Autodesk Fusion 360 part; units mm, degrees
(part 4 of 9)
  line L470 (39.3109, 74.8923) -> (43.641, 72.3923)
  line L471 (43.641, 72.3923) -> (47.9711, 74.8923)
  line L472 (47.9711, 74.8923) -> (47.9711, 79.8923)
  line L473 (47.9711, 79.8923) -> (43.641, 82.3923)
  line L474 (53.8013, 82.3923) -> (49.4711, 79.8923)
  line L475 (49.4711, 79.8923) -> (49.4711, 74.8923)
  line L476 (49.4711, 74.8923) -> (53.8013, 72.3923)
  line L477 (53.8013, 72.3923) -> (58.1314, 74.8923)
  line L478 (58.1314, 74.8923) -> (58.1314, 79.8923)
  line L479 (58.1314, 79.8923) -> (53.8013, 82.3923)
  line L480 (63.9615, 82.3923) -> (59.6314, 79.8923)
  line L481 (59.6314, 79.8923) -> (59.6314, 74.8923)
  line L482 (59.6314, 74.8923) -> (63.9615, 72.3923)
  line L483 (63.9615, 72.3923) -> (68.2917, 74.8923)
  line L484 (68.2917, 74.8923) -> (68.2917, 79.8923)
  line L485 (68.2917, 79.8923) -> (63.9615, 82.3923)
  line L486 (74.1218, 82.3923) -> (69.7917, 79.8923)
  line L487 (69.7917, 79.8923) -> (69.7917, 74.8923)
  line L488 (69.7917, 74.8923) -> (74.1218, 72.3923)
  line L489 (74.1218, 72.3923) -> (78.4519, 74.8923)
  line L490 (78.4519, 74.8923) -> (78.4519, 79.8923)
  line L491 (78.4519, 79.8923) -> (74.1218, 82.3923)
  line L492 (84.282, 82.3923) -> (79.9519, 79.8923)
  line L493 (79.9519, 79.8923) -> (79.9519, 74.8923)
  line L494 (79.9519, 74.8923) -> (84.282, 72.3923)
  line L495 (84.282, 72.3923) -> (88.6122, 74.8923)
  line L496 (88.6122, 74.8923) -> (88.6122, 79.8923)
  line L497 (88.6122, 79.8923) -> (84.282, 82.3923)
  line L498 (94.4423, 82.3923) -> (90.1122, 79.8923)
  line L499 (90.1122, 79.8923) -> (90.1122, 74.8923)
  line L500 (90.1122, 74.8923) -> (94.4423, 72.3923)
  line L501 (94.4423, 72.3923) -> (98.7724, 74.8923)
  line L502 (98.7724, 74.8923) -> (98.7724, 79.8923)
  line L503 (98.7724, 79.8923) -> (94.4423, 82.3923)
  line L504 (104.6025, 82.3923) -> (100.2724, 79.8923)
  line L505 (100.2724, 79.8923) -> (100.2724, 74.8923)
  line L506 (100.2724, 74.8923) -> (104.6025, 72.3923)
  line L507 (104.6025, 72.3923) -> (108.9327, 74.8923)
  line L508 (108.9327, 74.8923) -> (108.9327, 79.8923)
  line L509 (108.9327, 79.8923) -> (104.6025, 82.3923)
  line L510 (8.0801, 91.1913) -> (3.75, 88.6913)
  line L511 (3.75, 88.6913) -> (3.75, 83.6913)
  line L512 (3.75, 83.6913) -> (8.0801, 81.1913)
  line L513 (8.0801, 81.1913) -> (12.4103, 83.6913)
  line L514 (12.4103, 83.6913) -> (12.4103, 88.6913)
  line L515 (12.4103, 88.6913) -> (8.0801, 91.1913)
  line L516 (18.2404, 91.1913) -> (13.9103, 88.6913)
  line L517 (13.9103, 88.6913) -> (13.9103, 83.6913)
  line L518 (13.9103, 83.6913) -> (18.2404, 81.1913)
  line L519 (18.2404, 81.1913) -> (22.5705, 83.6913)
  line L520 (22.5705, 83.6913) -> (22.5705, 88.6913)
  line L521 (22.5705, 88.6913) -> (18.2404, 91.1913)
  line L522 (28.4006, 91.1913) -> (24.0705, 88.6913)
  line L523 (24.0705, 88.6913) -> (24.0705, 83.6913)
  line L524 (24.0705, 83.6913) -> (28.4006, 81.1913)
  line L525 (28.4006, 81.1913) -> (32.7308, 83.6913)
  line L526 (32.7308, 83.6913) -> (32.7308, 88.6913)
  line L527 (32.7308, 88.6913) -> (28.4006, 91.1913)
  line L528 (38.5609, 91.1913) -> (34.2308, 88.6913)
  line L529 (34.2308, 88.6913) -> (34.2308, 83.6913)
  line L530 (34.2308, 83.6913) -> (38.5609, 81.1913)
  line L531 (38.5609, 81.1913) -> (42.891, 83.6913)
  line L532 (42.891, 83.6913) -> (42.891, 88.6913)
  line L533 (42.891, 88.6913) -> (38.5609, 91.1913)
  line L534 (48.7211, 91.1913) -> (44.391, 88.6913)
  line L535 (44.391, 88.6913) -> (44.391, 83.6913)
  line L536 (44.391, 83.6913) -> (48.7211, 81.1913)
  line L537 (48.7211, 81.1913) -> (53.0513, 83.6913)
  line L538 (53.0513, 83.6913) -> (53.0513, 88.6913)
  line L539 (53.0513, 88.6913) -> (48.7211, 91.1913)
  line L540 (58.8814, 91.1913) -> (54.5513, 88.6913)
  line L541 (54.5513, 88.6913) -> (54.5513, 83.6913)
  line L542 (54.5513, 83.6913) -> (58.8814, 81.1913)
  line L543 (58.8814, 81.1913) -> (63.2115, 83.6913)
  line L544 (63.2115, 83.6913) -> (63.2115, 88.6913)
  line L545 (63.2115, 88.6913) -> (58.8814, 91.1913)
  line L546 (69.0417, 91.1913) -> (64.7115, 88.6913)
  line L547 (64.7115, 88.6913) -> (64.7115, 83.6913)
  line L548 (64.7115, 83.6913) -> (69.0417, 81.1913)
  line L549 (69.0417, 81.1913) -> (73.3718, 83.6913)
  line L550 (73.3718, 83.6913) -> (73.3718, 88.6913)
  line L551 (73.3718, 88.6913) -> (69.0417, 91.1913)
  line L552 (79.2019, 91.1913) -> (74.8718, 88.6913)
  line L553 (74.8718, 88.6913) -> (74.8718, 83.6913)
  line L554 (74.8718, 83.6913) -> (79.2019, 81.1913)
  line L555 (79.2019, 81.1913) -> (83.532, 83.6913)
  line L556 (83.532, 83.6913) -> (83.532, 88.6913)
  line L557 (83.532, 88.6913) -> (79.2019, 91.1913)
  line L558 (89.3622, 91.1913) -> (85.032, 88.6913)
  line L559 (85.032, 88.6913) -> (85.032, 83.6913)
  line L560 (85.032, 83.6913) -> (89.3622, 81.1913)
  line L561 (89.3622, 81.1913) -> (93.6923, 83.6913)
  line L562 (93.6923, 83.6913) -> (93.6923, 88.6913)
  line L563 (93.6923, 88.6913) -> (89.3622, 91.1913)
  line L564 (99.5224, 91.1913) -> (95.1923, 88.6913)
  line L565 (95.1923, 88.6913) -> (95.1923, 83.6913)
  line L566 (95.1923, 83.6913) -> (99.5224, 81.1913)
  line L567 (99.5224, 81.1913) -> (103.8525, 83.6913)
  line L568 (103.8525, 83.6913) -> (103.8525, 88.6913)
  line L569 (103.8525, 88.6913) -> (99.5224, 91.1913)
  line L570 (3, 99.9904) -> (-1.3301, 97.4904)
  line L571 (-1.3301, 97.4904) -> (-1.3301, 92.4904)
  line L572 (-1.3301, 92.4904) -> (3, 89.9904)
  line L573 (3, 89.9904) -> (7.3301, 92.4904)
  line L574 (7.3301, 92.4904) -> (7.3301, 97.4904)
  line L575 (7.3301, 97.4904) -> (3, 99.9904)
  line L576 (13.1603, 99.9904) -> (8.8301, 97.4904)
  line L577 (8.8301, 97.4904) -> (8.8301, 92.4904)
  line L578 (8.8301, 92.4904) -> (13.1603, 89.9904)
  line L579 (13.1603, 89.9904) -> (17.4904, 92.4904)
  line L580 (17.4904, 92.4904) -> (17.4904, 97.4904)
  line L581 (17.4904, 97.4904) -> (13.1603, 99.9904)
  line L582 (23.3205, 99.9904) -> (18.9904, 97.4904)
  line L583 (18.9904, 97.4904) -> (18.9904, 92.4904)
  line L584 (18.9904, 92.4904) -> (23.3205, 89.9904)
  line L585 (23.3205, 89.9904) -> (27.6506, 92.4904)
  line L586 (27.6506, 92.4904) -> (27.6506, 97.4904)
  line L587 (27.6506, 97.4904) -> (23.3205, 99.9904)
  line L588 (33.4808, 99.9904) -> (29.1506, 97.4904)
  line L589 (29.1506, 97.4904) -> (29.1506, 92.4904)
  line L590 (29.1506, 92.4904) -> (33.4808, 89.9904)
  line L591 (33.4808, 89.9904) -> (37.8109, 92.4904)
  line L592 (37.8109, 92.4904) -> (37.8109, 97.4904)
  line L593 (37.8109, 97.4904) -> (33.4808, 99.9904)
  line L594 (43.641, 99.9904) -> (39.3109, 97.4904)
  line L595 (39.3109, 97.4904) -> (39.3109, 92.4904)
  line L596 (39.3109, 92.4904) -> (43.641, 89.9904)
  line L597 (43.641, 89.9904) -> (47.9711, 92.4904)
  line L598 (47.9711, 92.4904) -> (47.9711, 97.4904)
  line L599 (47.9711, 97.4904) -> (43.641, 99.9904)
  line L600 (53.8013, 99.9904) -> (49.4711, 97.4904)
  line L601 (49.4711, 97.4904) -> (49.4711, 92.4904)
  line L602 (49.4711, 92.4904) -> (53.8013, 89.9904)
  line L603 (53.8013, 89.9904) -> (58.1314, 92.4904)
  line L604 (58.1314, 92.4904) -> (58.1314, 97.4904)
  line L605 (58.1314, 97.4904) -> (53.8013, 99.9904)
  line L606 (63.9615, 99.9904) -> (59.6314, 97.4904)
  line L607 (59.6314, 97.4904) -> (59.6314, 92.4904)
  line L608 (59.6314, 92.4904) -> (63.9615, 89.9904)
  line L609 (63.9615, 89.9904) -> (68.2917, 92.4904)
  line L610 (68.2917, 92.4904) -> (68.2917, 97.4904)
  line L611 (68.2917, 97.4904) -> (63.9615, 99.9904)
  line L612 (74.1218, 99.9904) -> (69.7917, 97.4904)
  line L613 (69.7917, 97.4904) -> (69.7917, 92.4904)
  line L614 (69.7917, 92.4904) -> (74.1218, 89.9904)
  line L615 (74.1218, 89.9904) -> (78.4519, 92.4904)
  line L616 (78.4519, 92.4904) -> (78.4519, 97.4904)
  line L617 (78.4519, 97.4904) -> (74.1218, 99.9904)
  line L618 (84.282, 99.9904) -> (79.9519, 97.4904)
  line L619 (79.9519, 97.4904) -> (79.9519, 92.4904)
  line L620 (79.9519, 92.4904) -> (84.282, 89.9904)
  line L621 (84.282, 89.9904) -> (88.6122, 92.4904)
  line L622 (88.6122, 92.4904) -> (88.6122, 97.4904)
  line L623 (88.6122, 97.4904) -> (84.282, 99.9904)
  line L624 (94.4423, 99.9904) -> (90.1122, 97.4904)
  line L625 (90.1122, 97.4904) -> (90.1122, 92.4904)
  line L626 (90.1122, 92.4904) -> (94.4423, 89.9904)
  line L627 (94.4423, 89.9904) -> (98.7724, 92.4904)
  line L628 (98.7724, 92.4904) -> (98.7724, 97.4904)
  line L629 (98.7724, 97.4904) -> (94.4423, 99.9904)
  line L630 (104.6025, 99.9904) -> (100.2724, 97.4904)
  line L631 (100.2724, 97.4904) -> (100.2724, 92.4904)
  line L632 (100.2724, 92.4904) -> (104.6025, 89.9904)
  line L633 (104.6025, 89.9904) -> (108.9327, 92.4904)
  line L634 (108.9327, 92.4904) -> (108.9327, 97.4904)
  line L635 (108.9327, 97.4904) -> (104.6025, 99.9904)
  line L636 (8.0801, 108.7894) -> (3.75, 106.2894)
  line L637 (3.75, 106.2894) -> (3.75, 101.2894)
  line L638 (3.75, 101.2894) -> (8.0801, 98.7894)
  line L639 (8.0801, 98.7894) -> (12.4103, 101.2894)
  line L640 (12.4103, 101.2894) -> (12.4103, 106.2894)
  line L641 (12.4103, 106.2894) -> (8.0801, 108.7894)
  line L642 (18.2404, 108.7894) -> (13.9103, 106.2894)
  line L643 (13.9103, 106.2894) -> (13.9103, 101.2894)
  line L644 (13.9103, 101.2894) -> (18.2404, 98.7894)
  line L645 (18.2404, 98.7894) -> (22.5705, 101.2894)
  line L646 (22.5705, 101.2894) -> (22.5705, 106.2894)
  line L647 (22.5705, 106.2894) -> (18.2404, 108.7894)
  line L648 (28.4006, 108.7894) -> (24.0705, 106.2894)
  line L649 (24.0705, 106.2894) -> (24.0705, 101.2894)
  line L650 (24.0705, 101.2894) -> (28.4006, 98.7894)
  line L651 (28.4006, 98.7894) -> (32.7308, 101.2894)
  line L652 (32.7308, 101.2894) -> (32.7308, 106.2894)
  line L653 (32.7308, 106.2894) -> (28.4006, 108.7894)
  line L654 (38.5609, 108.7894) -> (34.2308, 106.2894)
  line L655 (34.2308, 106.2894) -> (34.2308, 101.2894)
  line L656 (34.2308, 101.2894) -> (38.5609, 98.7894)
  line L657 (38.5609, 98.7894) -> (42.891, 101.2894)
  line L658 (42.891, 101.2894) -> (42.891, 106.2894)
  line L659 (42.891, 106.2894) -> (38.5609, 108.7894)
  line L660 (48.7211, 108.7894) -> (44.391, 106.2894)
  line L661 (44.391, 106.2894) -> (44.391, 101.2894)
  line L662 (44.391, 101.2894) -> (48.7211, 98.7894)
  line L663 (48.7211, 98.7894) -> (53.0513, 101.2894)
  line L664 (53.0513, 101.2894) -> (53.0513, 106.2894)
  line L665 (53.0513, 106.2894) -> (48.7211, 108.7894)
  line L666 (58.8814, 108.7894) -> (54.5513, 106.2894)
  line L667 (54.5513, 106.2894) -> (54.5513, 101.2894)
  line L668 (54.5513, 101.2894) -> (58.8814, 98.7894)
  line L669 (58.8814, 98.7894) -> (63.2115, 101.2894)
  line L670 (63.2115, 101.2894) -> (63.2115, 106.2894)
  line L671 (63.2115, 106.2894) -> (58.8814, 108.7894)
  line L672 (69.0417, 108.7894) -> (64.7115, 106.2894)
  line L673 (64.7115, 106.2894) -> (64.7115, 101.2894)
  line L674 (64.7115, 101.2894) -> (69.0417, 98.7894)
  line L675 (69.0417, 98.7894) -> (73.3718, 101.2894)
  line L676 (73.3718, 101.2894) -> (73.3718, 106.2894)
  line L677 (73.3718, 106.2894) -> (69.0417, 108.7894)
  line L678 (79.2019, 108.7894) -> (74.8718, 106.2894)
  line L679 (74.8718, 106.2894) -> (74.8718, 101.2894)
  line L680 (74.8718, 101.2894) -> (79.2019, 98.7894)
  line L681 (79.2019, 98.7894) -> (83.532, 101.2894)
  line L682 (83.532, 101.2894) -> (83.532, 106.2894)
  line L683 (83.532, 106.2894) -> (79.2019, 108.7894)
  line L684 (89.3622, 108.7894) -> (85.032, 106.2894)
  line L685 (85.032, 106.2894) -> (85.032, 101.2894)
  line L686 (85.032, 101.2894) -> (89.3622, 98.7894)
  line L687 (89.3622, 98.7894) -> (93.6923, 101.2894)
  line L688 (93.6923, 101.2894) -> (93.6923, 106.2894)
  line L689 (93.6923, 106.2894) -> (89.3622, 108.7894)
  line L690 (99.5224, 108.7894) -> (95.1923, 106.2894)
  line L691 (95.1923, 106.2894) -> (95.1923, 101.2894)
  line L692 (95.1923, 101.2894) -> (99.5224, 98.7894)
  line L693 (99.5224, 98.7894) -> (103.8525, 101.2894)
  line L694 (103.8525, 101.2894) -> (103.8525, 106.2894)
  line L695 (103.8525, 106.2894) -> (99.5224, 108.7894)
  line L696 (3, 117.5885) -> (-1.3301, 115.0885)
  line L697 (-1.3301, 115.0885) -> (-1.3301, 110.0885)
  line L698 (-1.3301, 110.0885) -> (3, 107.5885)
  line L699 (3, 107.5885) -> (7.3301, 110.0885)
  line L700 (7.3301, 110.0885) -> (7.3301, 115.0885)
  line L701 (7.3301, 115.0885) -> (3, 117.5885)
  line L702 (13.1603, 117.5885) -> (8.8301, 115.0885)
  line L703 (8.8301, 115.0885) -> (8.8301, 110.0885)
  line L704 (8.8301, 110.0885) -> (13.1603, 107.5885)
  line L705 (13.1603, 107.5885) -> (17.4904, 110.0885)
  line L706 (17.4904, 110.0885) -> (17.4904, 115.0885)
  line L707 (17.4904, 115.0885) -> (13.1603, 117.5885)
  line L708 (23.3205, 117.5885) -> (18.9904, 115.0885)
  line L709 (18.9904, 115.0885) -> (18.9904, 110.0885)
  line L710 (18.9904, 110.0885) -> (23.3205, 107.5885)
  line L711 (23.3205, 107.5885) -> (27.6506, 110.0885)
  line L712 (27.6506, 110.0885) -> (27.6506, 115.0885)
  line L713 (27.6506, 115.0885) -> (23.3205, 117.5885)
  line L714 (33.4808, 117.5885) -> (29.1506, 115.0885)
  line L715 (29.1506, 115.0885) -> (29.1506, 110.0885)
  line L716 (29.1506, 110.0885) -> (33.4808, 107.5885)
  line L717 (33.4808, 107.5885) -> (37.8109, 110.0885)
  line L718 (37.8109, 110.0885) -> (37.8109, 115.0885)
  line L719 (37.8109, 115.0885) -> (33.4808, 117.5885)
  line L720 (43.641, 117.5885) -> (39.3109, 115.0885)
  line L721 (39.3109, 115.0885) -> (39.3109, 110.0885)
  line L722 (39.3109, 110.0885) -> (43.641, 107.5885)
  line L723 (43.641, 107.5885) -> (47.9711, 110.0885)
  line L724 (47.9711, 110.0885) -> (47.9711, 115.0885)
  line L725 (47.9711, 115.0885) -> (43.641, 117.5885)
  line L726 (53.8013, 117.5885) -> (49.4711, 115.0885)
  line L727 (49.4711, 115.0885) -> (49.4711, 110.0885)
  line L728 (49.4711, 110.0885) -> (53.8013, 107.5885)
  line L729 (53.8013, 107.5885) -> (58.1314, 110.0885)
  line L730 (58.1314, 110.0885) -> (58.1314, 115.0885)
  line L731 (58.1314, 115.0885) -> (53.8013, 117.5885)
  line L732 (63.9615, 117.5885) -> (59.6314, 115.0885)
  line L733 (59.6314, 115.0885) -> (59.6314, 110.0885)
  line L734 (59.6314, 110.0885) -> (63.9615, 107.5885)
  line L735 (63.9615, 107.5885) -> (68.2917, 110.0885)
  line L736 (68.2917, 110.0885) -> (68.2917, 115.0885)
  line L737 (68.2917, 115.0885) -> (63.9615, 117.5885)
  line L738 (74.1218, 117.5885) -> (69.7917, 115.0885)
  line L739 (69.7917, 115.0885) -> (69.7917, 110.0885)
  line L740 (69.7917, 110.0885) -> (74.1218, 107.5885)
  line L741 (74.1218, 107.5885) -> (78.4519, 110.0885)
  line L742 (78.4519, 110.0885) -> (78.4519, 115.0885)
  line L743 (78.4519, 115.0885) -> (74.1218, 117.5885)
  line L744 (84.282, 117.5885) -> (79.9519, 115.0885)
  line L745 (79.9519, 115.0885) -> (79.9519, 110.0885)
  line L746 (79.9519, 110.0885) -> (84.282, 107.5885)
  line L747 (84.282, 107.5885) -> (88.6122, 110.0885)
  line L748 (88.6122, 110.0885) -> (88.6122, 115.0885)
  line L749 (88.6122, 115.0885) -> (84.282, 117.5885)
  line L750 (94.4423, 117.5885) -> (90.1122, 115.0885)
  line L751 (90.1122, 115.0885) -> (90.1122, 110.0885)
  line L752 (90.1122, 110.0885) -> (94.4423, 107.5885)
  line L753 (94.4423, 107.5885) -> (98.7724, 110.0885)
  line L754 (98.7724, 110.0885) -> (98.7724, 115.0885)
  line L755 (98.7724, 115.0885) -> (94.4423, 117.5885)
  line L756 (104.6025, 117.5885) -> (100.2724, 115.0885)
  line L757 (100.2724, 115.0885) -> (100.2724, 110.0885)
  line L758 (100.2724, 110.0885) -> (104.6025, 107.5885)
  line L759 (104.6025, 107.5885) -> (108.9327, 110.0885)
  line L760 (108.9327, 110.0885) -> (108.9327, 115.0885)
  line L761 (108.9327, 115.0885) -> (104.6025, 117.5885)
  line L762 (8.0801, 126.3875) -> (3.75, 123.8875)
  line L763 (3.75, 123.8875) -> (3.75, 118.8875)
  line L764 (3.75, 118.8875) -> (8.0801, 116.3875)
  line L765 (8.0801, 116.3875) -> (12.4103, 118.8875)
  line L766 (12.4103, 118.8875) -> (12.4103, 123.8875)
  line L767 (12.4103, 123.8875) -> (8.0801, 126.3875)
  line L768 (18.2404, 126.3875) -> (13.9103, 123.8875)
  line L769 (13.9103, 123.8875) -> (13.9103, 118.8875)
  line L770 (13.9103, 118.8875) -> (18.2404, 116.3875)
  line L771 (18.2404, 116.3875) -> (22.5705, 118.8875)
  line L772 (22.5705, 118.8875) -> (22.5705, 123.8875)
  line L773 (22.5705, 123.8875) -> (18.2404, 126.3875)
  line L774 (28.4006, 126.3875) -> (24.0705, 123.8875)
  line L775 (24.0705, 123.8875) -> (24.0705, 118.8875)
  line L776 (24.0705, 118.8875) -> (28.4006, 116.3875)
  line L777 (28.4006, 116.3875) -> (32.7308, 118.8875)
  line L778 (32.7308, 118.8875) -> (32.7308, 123.8875)
  line L779 (32.7308, 123.8875) -> (28.4006, 126.3875)
  line L780 (38.5609, 126.3875) -> (34.2308, 123.8875)
  line L781 (34.2308, 123.8875) -> (34.2308, 118.8875)
  line L782 (34.2308, 118.8875) -> (38.5609, 116.3875)
  line L783 (38.5609, 116.3875) -> (42.891, 118.8875)
  line L784 (42.891, 118.8875) -> (42.891, 123.8875)
  line L785 (42.891, 123.8875) -> (38.5609, 126.3875)
  line L786 (48.7211, 126.3875) -> (44.391, 123.8875)
  line L787 (44.391, 123.8875) -> (44.391, 118.8875)
  line L788 (44.391, 118.8875) -> (48.7211, 116.3875)
  line L789 (48.7211, 116.3875) -> (53.0513, 118.8875)
  line L790 (53.0513, 118.8875) -> (53.0513, 123.8875)
  line L791 (53.0513, 123.8875) -> (48.7211, 126.3875)
  line L792 (58.8814, 126.3875) -> (54.5513, 123.8875)
  line L793 (54.5513, 123.8875) -> (54.5513, 118.8875)
  line L794 (54.5513, 118.8875) -> (58.8814, 116.3875)
  line L795 (58.8814, 116.3875) -> (63.2115, 118.8875)
  line L796 (63.2115, 118.8875) -> (63.2115, 123.8875)
  line L797 (63.2115, 123.8875) -> (58.8814, 126.3875)
  line L798 (69.0417, 126.3875) -> (64.7115, 123.8875)
  line L799 (64.7115, 123.8875) -> (64.7115, 118.8875)
  line L800 (64.7115, 118.8875) -> (69.0417, 116.3875)
  line L801 (69.0417, 116.3875) -> (73.3718, 118.8875)
  line L802 (73.3718, 118.8875) -> (73.3718, 123.8875)
  line L803 (73.3718, 123.8875) -> (69.0417, 126.3875)
  line L804 (79.2019, 126.3875) -> (74.8718, 123.8875)
  line L805 (74.8718, 123.8875) -> (74.8718, 118.8875)
  line L806 (74.8718, 118.8875) -> (79.2019, 116.3875)
  line L807 (79.2019, 116.3875) -> (83.532, 118.8875)
  line L808 (83.532, 118.8875) -> (83.532, 123.8875)
  line L809 (83.532, 123.8875) -> (79.2019, 126.3875)
  line L810 (89.3622, 126.3875) -> (85.032, 123.8875)
  line L811 (85.032, 123.8875) -> (85.032, 118.8875)
  line L812 (85.032, 118.8875) -> (89.3622, 116.3875)
  line L813 (89.3622, 116.3875) -> (93.6923, 118.8875)
  line L814 (93.6923, 118.8875) -> (93.6923, 123.8875)
  line L815 (93.6923, 123.8875) -> (89.3622, 126.3875)
  line L816 (99.5224, 126.3875) -> (95.1923, 123.8875)
  line L817 (95.1923, 123.8875) -> (95.1923, 118.8875)
  line L818 (95.1923, 118.8875) -> (99.5224, 116.3875)
  line L819 (99.5224, 116.3875) -> (103.8525, 118.8875)
  line L820 (103.8525, 118.8875) -> (103.8525, 123.8875)
  line L821 (103.8525, 123.8875) -> (99.5224, 126.3875)
  line L822 (3, 135.1865) -> (-1.3301, 132.6865)
  line L823 (-1.3301, 132.6865) -> (-1.3301, 127.6865)
  line L824 (-1.3301, 127.6865) -> (3, 125.1865)
  line L825 (3, 125.1865) -> (7.3301, 127.6865)
  line L826 (7.3301, 127.6865) -> (7.3301, 132.6865)
  line L827 (7.3301, 132.6865) -> (3, 135.1865)
  line L828 (13.1603, 135.1865) -> (8.8301, 132.6865)
  line L829 (8.8301, 132.6865) -> (8.8301, 127.6865)
  line L830 (8.8301, 127.6865) -> (13.1603, 125.1865)
  line L831 (13.1603, 125.1865) -> (17.4904, 127.6865)
  line L832 (17.4904, 127.6865) -> (17.4904, 132.6865)
  line L833 (17.4904, 132.6865) -> (13.1603, 135.1865)
  line L834 (23.3205, 135.1865) -> (18.9904, 132.6865)
  line L835 (18.9904, 132.6865) -> (18.9904, 127.6865)
  line L836 (18.9904, 127.6865) -> (23.3205, 125.1865)
  line L837 (23.3205, 125.1865) -> (27.6506, 127.6865)
  line L838 (27.6506, 127.6865) -> (27.6506, 132.6865)
  line L839 (27.6506, 132.6865) -> (23.3205, 135.1865)
  line L840 (33.4808, 135.1865) -> (29.1506, 132.6865)
  line L841 (29.1506, 132.6865) -> (29.1506, 127.6865)
  line L842 (29.1506, 127.6865) -> (33.4808, 125.1865)
  line L843 (33.4808, 125.1865) -> (37.8109, 127.6865)
  line L844 (37.8109, 127.6865) -> (37.8109, 132.6865)
  line L845 (37.8109, 132.6865) -> (33.4808, 135.1865)
  line L846 (43.641, 135.1865) -> (39.3109, 132.6865)
  line L847 (39.3109, 132.6865) -> (39.3109, 127.6865)
  line L848 (39.3109, 127.6865) -> (43.641, 125.1865)
  line L849 (43.641, 125.1865) -> (47.9711, 127.6865)
  line L850 (47.9711, 127.6865) -> (47.9711, 132.6865)
  line L851 (47.9711, 132.6865) -> (43.641, 135.1865)
  line L852 (53.8013, 135.1865) -> (49.4711, 132.6865)
  line L853 (49.4711, 132.6865) -> (49.4711, 127.6865)
  line L854 (49.4711, 127.6865) -> (53.8013, 125.1865)
  line L855 (53.8013, 125.1865) -> (58.1314, 127.6865)
  line L856 (58.1314, 127.6865) -> (58.1314, 132.6865)
  line L857 (58.1314, 132.6865) -> (53.8013, 135.1865)
  line L858 (63.9615, 135.1865) -> (59.6314, 132.6865)
  line L859 (59.6314, 132.6865) -> (59.6314, 127.6865)
  line L860 (59.6314, 127.6865) -> (63.9615, 125.1865)
  line L861 (63.9615, 125.1865) -> (68.2917, 127.6865)
  line L862 (68.2917, 127.6865) -> (68.2917, 132.6865)
  line L863 (68.2917, 132.6865) -> (63.9615, 135.1865)
  line L864 (74.1218, 135.1865) -> (69.7917, 132.6865)
  line L865 (69.7917, 132.6865) -> (69.7917, 127.6865)
  line L866 (69.7917, 127.6865) -> (74.1218, 125.1865)
  line L867 (74.1218, 125.1865) -> (78.4519, 127.6865)
  line L868 (78.4519, 127.6865) -> (78.4519, 132.6865)
  line L869 (78.4519, 132.6865) -> (74.1218, 135.1865)
  line L870 (84.282, 135.1865) -> (79.9519, 132.6865)
  line L871 (79.9519, 132.6865) -> (79.9519, 127.6865)
  line L872 (79.9519, 127.6865) -> (84.282, 125.1865)
  line L873 (84.282, 125.1865) -> (88.6122, 127.6865)
  line L874 (88.6122, 127.6865) -> (88.6122, 132.6865)
  line L875 (88.6122, 132.6865) -> (84.282, 135.1865)
  line L876 (94.4423, 135.1865) -> (90.1122, 132.6865)
  line L877 (90.1122, 132.6865) -> (90.1122, 127.6865)
  line L878 (90.1122, 127.6865) -> (94.4423, 125.1865)
  line L879 (94.4423, 125.1865) -> (98.7724, 127.6865)
  line L880 (98.7724, 127.6865) -> (98.7724, 132.6865)
  line L881 (98.7724, 132.6865) -> (94.4423, 135.1865)
  line L882 (104.6025, 135.1865) -> (100.2724, 132.6865)
  line L883 (100.2724, 132.6865) -> (100.2724, 127.6865)
  line L884 (100.2724, 127.6865) -> (104.6025, 125.1865)
  line L885 (104.6025, 125.1865) -> (108.9327, 127.6865)
  line L886 (108.9327, 127.6865) -> (108.9327, 132.6865)
  line L887 (108.9327, 132.6865) -> (104.6025, 135.1865)
  line L888 (8.0801, 143.9856) -> (3.75, 141.4856)
  line L889 (3.75, 141.4856) -> (3.75, 136.4856)
  line L890 (3.75, 136.4856) -> (8.0801, 133.9856)
  line L891 (8.0801, 133.9856) -> (12.4103, 136.4856)
  line L892 (12.4103, 136.4856) -> (12.4103, 141.4856)
  line L893 (12.4103, 141.4856) -> (8.0801, 143.9856)
  line L894 (18.2404, 143.9856) -> (13.9103, 141.4856)
  line L895 (13.9103, 141.4856) -> (13.9103, 136.4856)
  line L896 (13.9103, 136.4856) -> (18.2404, 133.9856)
  line L897 (18.2404, 133.9856) -> (22.5705, 136.4856)
  line L898 (22.5705, 136.4856) -> (22.5705, 141.4856)
  line L899 (22.5705, 141.4856) -> (18.2404, 143.9856)
  line L900 (28.4006, 143.9856) -> (24.0705, 141.4856)
  line L901 (24.0705, 141.4856) -> (24.0705, 136.4856)
  line L902 (24.0705, 136.4856) -> (28.4006, 133.9856)
  line L903 (28.4006, 133.9856) -> (32.7308, 136.4856)
  line L904 (32.7308, 136.4856) -> (32.7308, 141.4856)
  line L905 (32.7308, 141.4856) -> (28.4006, 143.9856)
  line L906 (38.5609, 143.9856) -> (34.2308, 141.4856)
  line L907 (34.2308, 141.4856) -> (34.2308, 136.4856)
  line L908 (34.2308, 136.4856) -> (38.5609, 133.9856)
  line L909 (38.5609, 133.9856) -> (42.891, 136.4856)
  line L910 (42.891, 136.4856) -> (42.891, 141.4856)
  line L911 (42.891, 141.4856) -> (38.5609, 143.9856)
  line L912 (48.7211, 143.9856) -> (44.391, 141.4856)
  line L913 (44.391, 141.4856) -> (44.391, 136.4856)
  line L914 (44.391, 136.4856) -> (48.7211, 133.9856)
  line L915 (48.7211, 133.9856) -> (53.0513, 136.4856)
  line L916 (53.0513, 136.4856) -> (53.0513, 141.4856)
  line L917 (53.0513, 141.4856) -> (48.7211, 143.9856)
  line L918 (58.8814, 143.9856) -> (54.5513, 141.4856)
  line L919 (54.5513, 141.4856) -> (54.5513, 136.4856)
  line L920 (54.5513, 136.4856) -> (58.8814, 133.9856)
  line L921 (58.8814, 133.9856) -> (63.2115, 136.4856)
  line L922 (63.2115, 136.4856) -> (63.2115, 141.4856)
  line L923 (63.2115, 141.4856) -> (58.8814, 143.9856)
  line L924 (69.0417, 143.9856) -> (64.7115, 141.4856)
  line L925 (64.7115, 141.4856) -> (64.7115, 136.4856)
  line L926 (64.7115, 136.4856) -> (69.0417, 133.9856)
  line L927 (69.0417, 133.9856) -> (73.3718, 136.4856)
  line L928 (73.3718, 136.4856) -> (73.3718, 141.4856)
  line L929 (73.3718, 141.4856) -> (69.0417, 143.9856)
  line L930 (79.2019, 143.9856) -> (74.8718, 141.4856)
  line L931 (74.8718, 141.4856) -> (74.8718, 136.4856)
  line L932 (74.8718, 136.4856) -> (79.2019, 133.9856)
  line L933 (79.2019, 133.9856) -> (83.532, 136.4856)
  line L934 (83.532, 136.4856) -> (83.532, 141.4856)
  line L935 (83.532, 141.4856) -> (79.2019, 143.9856)
  line L936 (89.3622, 143.9856) -> (85.032, 141.4856)
  line L937 (85.032, 141.4856) -> (85.032, 136.4856)
  line L938 (85.032, 136.4856) -> (89.3622, 133.9856)
  line L939 (89.3622, 133.9856) -> (93.6923, 136.4856)
  line L940 (93.6923, 136.4856) -> (93.6923, 141.4856)
  line L941 (93.6923, 141.4856) -> (89.3622, 143.9856)
  line L942 (99.5224, 143.9856) -> (95.1923, 141.4856)
  line L943 (95.1923, 141.4856) -> (95.1923, 136.4856)
  line L944 (95.1923, 136.4856) -> (99.5224, 133.9856)
  line L945 (99.5224, 133.9856) -> (103.8525, 136.4856)
  line L946 (103.8525, 136.4856) -> (103.8525, 141.4856)
  line L947 (103.8525, 141.4856) -> (99.5224, 143.9856)
  line L948 (3, 152.7846) -> (-1.3301, 150.2846)
  line L949 (-1.3301, 150.2846) -> (-1.3301, 145.2846)
  line L950 (-1.3301, 145.2846) -> (3, 142.7846)
  line L951 (3, 142.7846) -> (7.3301, 145.2846)
  line L952 (7.3301, 145.2846) -> (7.3301, 150.2846)
  line L953 (7.3301, 150.2846) -> (3, 152.7846)
  line L954 (13.1603, 152.7846) -> (8.8301, 150.2846)
  line L955 (8.8301, 150.2846) -> (8.8301, 145.2846)
  line L956 (8.8301, 145.2846) -> (13.1603, 142.7846)
  line L957 (13.1603, 142.7846) -> (17.4904, 145.2846)
  line L958 (17.4904, 145.2846) -> (17.4904, 150.2846)
  line L959 (17.4904, 150.2846) -> (13.1603, 152.7846)
  line L960 (23.3205, 152.7846) -> (18.9904, 150.2846)
  line L961 (18.9904, 150.2846) -> (18.9904, 145.2846)
  line L962 (18.9904, 145.2846) -> (23.3205, 142.7846)
  line L963 (23.3205, 142.7846) -> (27.6506, 145.2846)
  line L964 (27.6506, 145.2846) -> (27.6506, 150.2846)
  line L965 (27.6506, 150.2846) -> (23.3205, 152.7846)
  line L966 (33.4808, 152.7846) -> (29.1506, 150.2846)
  line L967 (29.1506, 150.2846) -> (29.1506, 145.2846)
  line L968 (29.1506, 145.2846) -> (33.4808, 142.7846)
  line L969 (33.4808, 142.7846) -> (37.8109, 145.2846)
  line L970 (37.8109, 145.2846) -> (37.8109, 150.2846)
  line L971 (37.8109, 150.2846) -> (33.4808, 152.7846)
  line L972 (43.641, 152.7846) -> (39.3109, 150.2846)
  line L973 (39.3109, 150.2846) -> (39.3109, 145.2846)
  line L974 (39.3109, 145.2846) -> (43.641, 142.7846)
  line L975 (43.641, 142.7846) -> (47.9711, 145.2846)
  line L976 (47.9711, 145.2846) -> (47.9711, 150.2846)
  line L977 (47.9711, 150.2846) -> (43.641, 152.7846)
  line L978 (53.8013, 152.7846) -> (49.4711, 150.2846)
  line L979 (49.4711, 150.2846) -> (49.4711, 145.2846)
  line L980 (49.4711, 145.2846) -> (53.8013, 142.7846)
  line L981 (53.8013, 142.7846) -> (58.1314, 145.2846)
  line L982 (58.1314, 145.2846) -> (58.1314, 150.2846)
  line L983 (58.1314, 150.2846) -> (53.8013, 152.7846)
  line L984 (63.9615, 152.7846) -> (59.6314, 150.2846)
  line L985 (59.6314, 150.2846) -> (59.6314, 145.2846)
  line L986 (59.6314, 145.2846) -> (63.9615, 142.7846)
  line L987 (63.9615, 142.7846) -> (68.2917, 145.2846)
  line L988 (68.2917, 145.2846) -> (68.2917, 150.2846)
  line L989 (68.2917, 150.2846) -> (63.9615, 152.7846)
  line L990 (74.1218, 152.7846) -> (69.7917, 150.2846)
  line L991 (69.7917, 150.2846) -> (69.7917, 145.2846)
  line L992 (69.7917, 145.2846) -> (74.1218, 142.7846)
  line L993 (74.1218, 142.7846) -> (78.4519, 145.2846)
  line L994 (78.4519, 145.2846) -> (78.4519, 150.2846)
  line L995 (78.4519, 150.2846) -> (74.1218, 152.7846)
  line L996 (84.282, 152.7846) -> (79.9519, 150.2846)
  line L997 (79.9519, 150.2846) -> (79.9519, 145.2846)
  line L998 (79.9519, 145.2846) -> (84.282, 142.7846)
  line L999 (84.282, 142.7846) -> (88.6122, 145.2846)
  line L1000 (88.6122, 145.2846) -> (88.6122, 150.2846)
  line L1001 (88.6122, 150.2846) -> (84.282, 152.7846)
  line L1002 (94.4423, 152.7846) -> (90.1122, 150.2846)
  line L1003 (90.1122, 150.2846) -> (90.1122, 145.2846)
  line L1004 (90.1122, 145.2846) -> (94.4423, 142.7846)
  line L1005 (94.4423, 142.7846) -> (98.7724, 145.2846)
  line L1006 (98.7724, 145.2846) -> (98.7724, 150.2846)
  line L1007 (98.7724, 150.2846) -> (94.4423, 152.7846)
  line L1008 (104.6025, 152.7846) -> (100.2724, 150.2846)
  line L1009 (100.2724, 150.2846) -> (100.2724, 145.2846)
  line L1010 (100.2724, 145.2846) -> (104.6025, 142.7846)
  line L1011 (104.6025, 142.7846) -> (108.9327, 145.2846)
  line L1012 (108.9327, 145.2846) -> (108.9327, 150.2846)
  line L1013 (108.9327, 150.2846) -> (104.6025, 152.7846)
extrude "拉伸23" cut sketch "草图22" against normal blind 5 contours L6 L7 L8 L9 L10 L11 | L12 L13 L14 L15 L16 L17 | L18 L19 L20 L21 L22 L23 | L24 L25 L26 L27 L28 L29 | L30 L31 L32 L33 L34 L35 | L36 L37 L38 L39 L40 L41 | L42 L43 L44 L45 L46 L47 | L48 L49 L50 L51 L52 L53 | L54 L55 L56 L57 L58 L59 | L60 L61 L62 L63 L64 L65 | L66 L67 L68 L69 L70 L71 | L72 L73 L74 L75 L76 L77 | L78 L79 L80 L81 L82 L83 | L84 L85 L86 L87 L88 L89 | L90 L91 L92 L93 L94 L95 | L96 L97 L98 L99 L100 L101 | L102 L103 L104 L105 L106 L107 | L108 L109 L110 L111 L112 L113 | L114 L115 L116 L117 L118 L119 | L120 L121 L122 L123 L124 L125 | L126 L127 L128 L129 L130 L131 | L132 L133 L134 L135 L136 L137 | L138 L139 L140 L141 L142 L143 | L144 L145 L146 L147 L148 L149 | L150 L151 L152 L153 L154 L155 | L156 L157 L158 L159 L160 L161 | L162 L163 L164 L165 L166 L167 | L168 L169 L170 L171 L172 L173 | L174 L175 L176 L177 L178 L179 | L180 L181 L182 L183 L184 L185 | L186 L187 L188 L189 L190 L191 | L192 L193 L194 L195 L196 L197 | L198 L199 L200 L201 L202 L203 | L204 L205 L206 L207 L208 L209 | L210 L211 L212 L213 L214 L215 | L216 L217 L218 L219 L220 L221 | L222 L223 L224 L225 L226 L227 | L228 L229 L230 L231 L232 L233 | L234 L235 L236 L237 L238 L239 | L240 L241 L242 L243 L244 L245 | L246 L247 L248 L249 L250 L251 | L252 L253 L254 L255 L256 L257 | L258 L259 L260 L261 L262 L263 | L264 L265 L266 L267 L268 L269 | L270 L271 L272 L273 L274 L275 | L276 L277 L278 L279 L280 L281 | L282 L283 L284 L285 L286 L287 | L288 L289 L290 L291 L292 L293 | L294 L295 L296 L297 L298 L299 | L300 L301 L302 L303 L304 L305 | L306 L307 L308 L309 L310 L311 | L312 L313 L314 L315 L316 L317 | L318 L319 L320 L321 L322 L323 | L324 L325 L326 L327 L328 L329 | L330 L331 L332 L333 L334 L335 | L336 L337 L338 L339 L340 L341 | L342 L343 L344 L345 L346 L347 | L348 L349 L350 L351 L352 L353 | L354 L355 L356 L357 L358 L359 | L360 L361 L362 L363 L364 L365 | L366 L367 L368 L369 L370 L371 | L372 L373 L374 L375 L376 L377 | L378 L379 L380 L381 L382 L383 | L384 L385 L386 L387 L388 L389 | L390 L391 L392 L393 L394 L395 | L396 L397 L398 L399 L400 L401 | L402 L403 L404 L405 L406 L407 | L408 L409 L410 L411 L412 L413 | L414 L415 L416 L417 L418 L419 | L420 L421 L422 L423 L424 L425 | L426 L427 L428 L429 L430 L431 | L432 L433 L434 L435 L436 L437 | L438 L439 L440 L441 L442 L443 | L444 L445 L446 L447 L448 L449 | L450 L451 L452 L453 L454 L455 | L456 L457 L458 L459 L460 L461 | L462 L463 L464 L465 L466 L467 | L468 L469 L470 L471 L472 L473 | L474 L475 L476 L477 L478 L479 | L480 L481 L482 L483 L484 L485 | L486 L487 L488 L489 L490 L491 | L492 L493 L494 L495 L496 L497 | L498 L499 L500 L501 L502 L503 | L504 L505 L506 L507 L508 L509 | L510 L511 L512 L513 L514 L515 | L516 L517 L518 L519 L520 L521 | L522 L523 L524 L525 L526 L527 | L528 L529 L530 L531 L532 L533 | L534 L535 L536 L537 L538 L539 | L540 L541 L542 L543 L544 L545 | L546 L547 L548 L549 L550 L551 | L552 L553 L554 L555 L556 L557 | L558 L559 L560 L561 L562 L563 | L564 L565 L566 L567 L568 L569 | L570 L571 L572 L573 L574 L575 | L576 L577 L578 L579 L580 L581 | L582 L583 L584 L585 L586 L587 | L588 L589 L590 L591 L592 L593 | L594 L595 L596 L597 L598 L599 | L600 L601 L602 L603 L604 L605 | L606 L607 L608 L609 L610 L611 | L612 L613 L614 L615 L616 L617 | L618 L619 L620 L621 L622 L623 | L624 L625 L626 L627 L628 L629 | L630 L631 L632 L633 L634 L635 | L636 L637 L638 L639 L640 L641 | L642 L643 L644 L645 L646 L647 | L648 L649 L650 L651 L652 L653 | L654 L655 L656 L657 L658 L659 | L660 L661 L662 L663 L664 L665 | L666 L667 L668 L669 L670 L671 | L672 L673 L674 L675 L676 L677 | L678 L679 L680 L681 L682 L683 | L684 L685 L686 L687 L688 L689 | L690 L691 L692 L693 L694 L695 | L696 L697 L698 L699 L700 L701 | L702 L703 L704 L705 L706 L707 | L708 L709 L710 L711 L712 L713 | L714 L715 L716 L717 L718 L719 | L720 L721 L722 L723 L724 L725 | L726 L727 L728 L729 L730 L731 | L732 L733 L734 L735 L736 L737 | L738 L739 L740 L741 L742 L743 | L744 L745 L746 L747 L748 L749 | L750 L751 L752 L753 L754 L755 | L756 L757 L758 L759 L760 L761 | L762 L763 L764 L765 L766 L767 | L768 L769 L770 L771 L772 L773 | L774 L775 L776 L777 L778 L779 | L780 L781 L782 L783 L784 L785 | L786 L787 L788 L789 L790 L791 | L792 L793 L794 L795 L796 L797 | L798 L799 L800 L801 L802 L803 | L804 L805 L806 L807 L808 L809 | L810 L811 L812 L813 L814 L815 | L816 L817 L818 L819 L820 L821 | L822 L823 L824 L825 L826 L827 | L828 L829 L830 L831 L832 L833 | L834 L835 L836 L837 L838 L839 | L840 L841 L842 L843 L844 L845 | L846 L847 L848 L849 L850 L851 | L852 L853 L854 L855 L856 L857 | L858 L859 L860 L861 L862 L863 | L864 L865 L866 L867 L868 L869 | L870 L871 L872 L873 L874 L875 | L876 L877 L878 L879 L880 L881 | L882 L883 L884 L885 L886 L887 | L888 L889 L890 L891 L892 L893 | L894 L895 L896 L897 L898 L899 | L900 L901 L902 L903 L904 L905 | L906 L907 L908 L909 L910 L911 | L912 L913 L914 L915 L916 L917 | L918 L919 L920 L921 L922 L923 | L924 L925 L926 L927 L928 L929 | L930 L931 L932 L933 L934 L935 | L936 L937 L938 L939 L940 L941 | L942 L943 L944 L945 L946 L947 | L948 L949 L950 L951 L952 L953 | L954 L955 L956 L957 L958 L959 | L960 L961 L962 L963 L964 L965 | L966 L967 L968 L969 L970 L971 | L972 L973 L974 L975 L976 L977 | L978 L979 L980 L981 L982 L983 | L984 L985 L986 L987 L988 L989 | L990 L991 L992 L993 L994 L995 | L996 L997 L998 L999 L1000 L1001 | L1002 L1003 L1004 L1005 L1006 L1007 | L1008 L1009 L1010 L1011 L1012 L1013 bodies 1